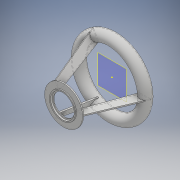
# Autodesk Inventor part: sizing_demo_magnet_holder
Saved by Autodesk Inventor 2018 (Build 220112000, 112)
## iProperties
Created: 2026-04-29
Part Number: sizing_demo_magnet_holder
Material: Generic
Document SubType Name: Modeling
Designer: neo
Density: 1 g/cm^3
Appearance: Default
Author: neo
Autodesk Inventor part; units mm, degrees
ref_plane "YZ Plane" through (0, 0, 0) normal (1, 0, 0) x (0, 1, 0)
ref_plane "XZ Plane" through (0, 0, 0) normal (0, 1, 0) x (-1, 0, 0)
ref_plane "XY Plane" through (0, 0, 0) normal (0, 0, 1) x (1, 0, 0)
sketch "Sketch1" plane through (0, 0, 0) normal (0, 1, 0) x (-1, 0, 0)
  circle A0 centre (0, 0) radius 50
  circle A1 centre (0, 0) radius 55
  dimension "d0" = 100
  dimension "d1" = 110
  constraints: 2 centre point, 2 coincident
  measures "d0" diameter of A0
  measures "d1" diameter of A1
extrude "Extrusion1" add sketch "Sketch1" along normal blind 10
sketch "Sketch2" plane through (0, 10, 0) normal (0, 1, 0) x (1, 0, 0)
  circle A0 centre (0, 0) radius 45
  circle A1 centre (0, 0) radius 50 projected
  dimension "d4" = 5
  constraints: 1 centre point, 1 coincident
  measures "d4" radial gap between concentric circles of A0 A1
extrude "Extrusion2" add sketch "Sketch2" against normal blind 3
ref_plane "200mm offset" through (0, 210, 0) normal (0, 1, 0) x (1, 0, 0)
sketch "Sketch4" plane through (0, 0, 0) normal (0, 0, 1) x (1, 0, 0)
  line L0 (-98.65, 210) -> (206.9, 210) projected
  line L1 (55, 10) -> (-55, 10) projected
  line L2 (0, 10) -> (0, 277.9846)
  circle A0 centre (140, 210) radius 20.25
  circle A1 centre (140, 210) radius 23.25
  point P0 (0, 0)
  dimension "d8" = 280
  dimension "d9" = 40.5
  dimension "d10" = 3
  constraints: 2 centre point, 2 end point, 1 coincident, 1 midpoint, 1 point on line, 1 vertical
  measures "d8" diameter of A0.centre L2
  measures "d9" diameter of A0
  measures "d10" radial gap between concentric circles of A0 A1
revolve "Revolution1" add sketch "Sketch4" angle 360 about axis through (0, 10, 0) along (0, 1, 0) contours A0 L0 A1 | L0 A1 A0
sketch "Sketch5" plane through (0, 10, 0) normal (0, 1, 0) x (1, 0, 0)
  circle A0 centre (0, 0) radius 80
  circle A1 centre (0, 0) radius 55 projected
  dimension "d12" = 25
  constraints: 1 centre point, 1 coincident
  measures "d12" radial gap between concentric circles of A0 A1
extrude "Extrusion3" add sketch "Sketch5" against normal blind 5
sketch "Sketch6" plane through (0, 210, 0) normal (0, 1, 0) x (1, 0, 0)
  point P0 (0, 0)
sketch "Sketch7" plane through (0, 0, 0) normal (0, 0, 1) x (1, 0, 0)
  arc A0 (140, 230.25) -> (140, 189.75) centre (140, 210) ccw construction
  arc A1 (140, 186.75) -> (140, 233.25) centre (140, 210) ccw construction
  line L0 (116.75, 210) -> (163.25, 210)
  line L1 (-80, 5) -> (80, 5) construction
  line L2 (-80, 10) -> (80, 10) construction
  line L3 (-45, 10) -> (45, 10) projected
  line L4 (45, 10) -> (116.75, 210)
  line L5 (163.25, 210) -> (80, 10)
  line L6 (45, 10) -> (80, 10)
  line L7 (45, 7) -> (-45, 7) projected
  point P0 (0, 0)
  constraints: 8 end point, 1 parallel, 1 point on circle
extrude "Extrusion4" add sketch "Sketch7" along normal mid plane 5
pattern_circular "Circular Pattern1" count 3 over 360 about axis through (0, 10, 0) along (0, -1, 0) of "Extrusion4"
body "Solid1"
